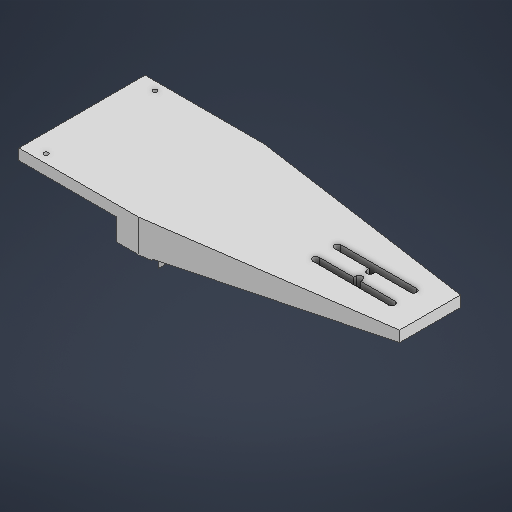
# Autodesk Inventor part: X Axis Vertical Snake Toolhead
Saved by Autodesk Inventor 2026 (Build 300175000, 175)
## iProperties
Created: 2025-04-17
Part Number: X Axis Vertical Snake Toolhead
Material: Generic
Document SubType Name: Modeling
Designer: lucse
Density: 1 g/cm^3
Appearance: Default
Author: lucse
Autodesk Inventor part; units mm, degrees
ref_plane "YZ Plane" through (0, 0, 0) normal (1, 0, 0) x (0, 1, 0)
ref_plane "XZ Plane" through (0, 0, 0) normal (0, 1, 0) x (-1, 0, 0)
ref_plane "XY Plane" through (0, 0, 0) normal (0, 0, 1) x (1, 0, 0)
sketch "Sketch1" plane through (0, 0, 0) normal (0, 1, 0) x (-1, 0, 0)
  line L0 (0, 29) -> (-160, 29)
  line L1 (-160, 29) -> (-160, -29)
  line L2 (-160, -29) -> (0, -29)
  line L3 (0, -29) -> (0, 29)
  point P0 (0, 0)
  point P1 (0, 0)
  dimension "d0" = 160
  dimension "d1" = 58
  constraints: 8 end point, 2 coincident, 2 parallel, 1 horizontal, 1 midpoint, 1 perpendicular
  measures "d0" distance of L1.end L2.end
  measures "d1" distance of L0.end L1.end
extrude "Extrusion1" add sketch "Sketch1" along normal blind 5
sketch "Sketch2" plane through (0, 5, 0) normal (0, 1, 0) x (1, 0, 0)
  circle A0 centre (8.5, -25) radius 1
  circle A1 centre (8.5, 25) radius 1
  line L0 (0, -29) -> (160, -29) projected
  line L1 (160, 29) -> (0, 29) projected
  line L2 (0, 29) -> (0, -29) projected
  line L3 (8.5, 25) -> (8.5, -25) construction
  line L4 (8.5, 0) -> (0, 0) construction
  dimension "d4" = 2
  dimension "d5" = 2
  dimension "d9" = 50
  dimension "d19" = 8.5
  constraints: 4 end point, 2 centre point, 1 horizontal, 1 midpoint, 1 vertical
  measures "d4" diameter of A0
  measures "d5" diameter of A1
  measures "d9" distance of L3.start L3.end
  measures "d19" distance from line of L2 L3.start
extrude "Extrusion2" cut sketch "Sketch2" against normal blind 6
sketch "Sketch4" plane through (0, 0, 0) normal (0, -1, 0) x (1, 0, 0)
  circle A0 centre (8.5, 25) radius 1 projected
  line L0 (160, 29) -> (160, -29) projected
  line L1 (0, 29) -> (160, 29) projected
  line L2 (0, -29) -> (0, 29) projected
  line L3 (160, -29) -> (0, -29) projected
  line L4 (45, 29) -> (45, -29)
  line L5 (53, 29) -> (53, -29)
  point P0 (0, 0)
  dimension "d18" = 45
  dimension "d20" = 8
  constraints: 4 end point, 4 point on line, 2 perpendicular
  measures "d18" distance between parallel lines of L2 L4
  measures "d20" distance between parallel lines of L4 L5
extrude "Extrusion3" add sketch "Sketch4" along normal blind 10 contours L5 L3 L4 L1
chamfer "Chamfer1" distance 107 distance2 10 1 edges at (53, 0, 0) measured on face at (53.5, 0, 0)
sketch "Sketch5" plane through (0, 5, 0) normal (0, 1, 0) x (1, 0, 0)
  line L0 (131.5, -3.5) -> (131.5, 3.5)
  line L1 (130, -3.5) -> (130, 3.5) construction
  line L2 (147.5, 3.5) -> (112.5, 3.5)
  line L3 (112.5, 6.5) -> (147.5, 6.5)
  line L4 (147.5, -6.5) -> (112.5, -6.5)
  line L5 (125, 3.5) -> (125, -3.5)
  line L6 (128.5, 3.5) -> (128.5, -3.5)
  circle A0 centre (147.5, 5) radius 1.5
  circle A1 centre (112.5, 5) radius 1.5
  circle A2 centre (112.5, -5) radius 1.5
  line L7 (112.5, -3.5) -> (147.5, -3.5)
  circle A3 centre (147.5, -5) radius 1.5
  line L8 (135, -3.5) -> (135, 3.5)
  line L9 (130, -3.5) -> (130, -15.5) construction
  line L10 (128.5, 1) -> (131.5, 1)
  line L11 (131.5, -1) -> (128.5, -1)
  circle A4 centre (8.5, -25) radius 1 projected
  line L12 (160, -29) -> (160, 29) projected
  line L13 (160, 29) -> (0, 29) projected
  line L14 (0, 29) -> (0, -29) projected
  line L15 (0, -29) -> (160, -29) projected
  line L16 (135, 0) -> (160, 0) construction
  point P0 (0, 0)
  point P1 (130, 0)
  point P2 (130, 1)
  dimension "d26" = 3
  dimension "d27" = 35
  dimension "d28" = 7
  dimension "d29" = 3
  dimension "d30" = 35
  dimension "d31" = 5
  dimension "d32" = 5
  dimension "d33" = 12
  dimension "d34" = 3
  dimension "d35" = 1.5
  dimension "d36" = 2
  dimension "d37" = 1
  dimension "d38" = 25
  constraints: 26 end point, 12 point on line, 8 point on circle, 8 tangent, 6 midpoint, 6 perpendicular, 4 centre point, 3 horizontal, 2 equal radius, 2 vertical
  measures "d26" diameter of A1
  measures "d27" distance of L3.start L3.end
  measures "d28" distance of L1.start L1.end
  measures "d29" diameter of A2
  measures "d30" distance of L7.start L7.end
  measures "d31" distance between parallel lines of L5 L1
  measures "d32" distance between parallel lines of L1 L8
  measures "d33" distance of L1.start L9.end
  measures "d34" distance between parallel lines of L0 L6
  measures "d35" distance between parallel lines of L1 L6
  measures "d36" distance between parallel lines of L11 L10
  measures "d37" distance of point (130, 0) point (130, 1)
  measures "d38" distance of L16.start L16.end
extrude "Extrusion4" cut sketch "Sketch5" against normal through all contours L7 L6 L11 L0 | L7 A3 L4 A2 | L10 L6 L2 L0 | A3 | L2 A1 L3 A0 | A2 | A0 | A1
fillet "Fillet1" radius 1.5 4 edges at (128.5, 1.0281, 1) (131.5, 1.1683, 1) (128.5, 1.0281, -1) (131.5, 1.1683, -1)
chamfer "Chamfer2" distance 105 distance2 15 1 edges at (160, 2.5, 29) measured on face at (159.5, 2.5, 29)
chamfer "Chamfer3" distance 105 distance2 15 1 edges at (160, 2.5, -29) measured on face at (159.5, 2.5, -29)
sketch "Sketch6" plane through (0, -10, 0) normal (0, -1, 0) x (1, 0, 0)
  line L0 (53, 29) -> (45, 29) projected
  line L1 (45, 29) -> (45, -29) projected
  line L2 (45, -29) -> (53, -29) projected
  line L3 (53, -29) -> (53, 29) projected
  line L4 (45, 10) -> (53, 10)
  line L5 (45, -10) -> (53, -10)
  line L6 (45, 29) -> (45, -29) projected
  point P0 (0, 0)
  point P1 (45, 0)
  point P2 (45, 0)
  dimension "d48" = 10
  dimension "d49" = 10
  constraints: 4 end point, 4 point on line, 2 midpoint, 2 perpendicular
  measures "d48" distance from line of point (45, 0) L4
  measures "d49" distance from line of point (45, 0) L5
extrude "Extrusion5" add sketch "Sketch6" along normal blind 20 contours L3 L5 L1 L4
fillet "Fillet2" radius 5 2 edges at (49, -10, 10) (49, -10, -10)
chamfer "Chamfer4" distance 8 angle 45 2 edges at (53, -30, 0) (53, -9.9999, 0)
sketch "Sketch7" plane through (160, 0, -14) normal (0.0930524, -0.9956612, 0) x (0.9956612, 0.0930524, 0)
  line L0 (-52.6307, 24) -> (-7.6307, 24)
  line L1 (-7.6307, 24) -> (-7.6307, 4)
  line L2 (-7.6307, 4) -> (-52.6307, 4)
  line L3 (-52.6307, 4) -> (-52.6307, 24)
  ellipse E0 centre (-30.1307, 16.5) end of major axis (-31.6373, 16.5) minor radius 1.5 (-31.6373, 16.5) -> (-28.6242, 16.5) ccw construction
  ellipse E1 centre (-30.1307, 11.5) end of major axis (-28.6242, 11.5) minor radius 1.5 (-28.6242, 11.5) -> (-31.6373, 11.5) ccw construction
  line L4 (-30.1307, 16.5) -> (-30.1307, 11.5) construction
  line L5 (-30.1307, 14) -> (-52.6307, 14) construction
  line L6 (-30.1307, 14) -> (-7.6307, 14) construction
  point P0 (-159.3058, 14)
  dimension "d56" = 20
  dimension "d57" = 45
  constraints: 14 end point, 3 midpoint, 2 horizontal, 2 parallel, 1 collinear, 1 perpendicular, 1 vertical, 2 other
  measures "d56" distance of L2.end L0.start
  measures "d57" distance of L0.start L0.end
extrude "Extrusion6" cut sketch "Sketch7" along normal blind 20 starts on plane at (80, 0, 0) facing (0, 1, 0)
equation "\"d32\" = d31"
equation "\"d35\" = 0.5 * d34"
equation "\"d37\" = 0.5 * d36"
equation "\"d49\" = d48"
body "Solid1"
